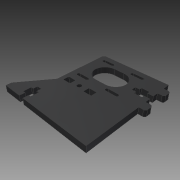
# Autodesk Inventor part: y_motor_mount
Saved by Autodesk Inventor 2014 (Build 180170000, 170)
## iProperties
Created: 2013-12-07
Part Number: y_motor_mount
Material: Generic
Document SubType Name: Modeling
Designer: buben
Density: 1 g/cm^3
Appearance: Anodized - Dark Gray
Author: buben
Subject: Laser Cutted
Autodesk Inventor part; units mm, degrees
ref_plane "YZ Plane" through (0, 0, 0) normal (1, 0, 0) x (0, 1, 0)
ref_plane "XZ Plane" through (0, 0, 0) normal (0, 1, 0) x (-1, 0, 0)
ref_plane "XY Plane" through (0, 0, 0) normal (0, 0, 1) x (1, 0, 0)
sketch "Sketch1" plane through (0, 0, 0) normal (0, 0, 1) x (1, 0, 0)
  line L0 (0, 0) -> (67.3, 0)
  line L1 (67.3, 0) -> (67.3, 55)
  line L2 (67.3, 55) -> (0, 55)
  line L3 (0, 55) -> (0, 0)
  line L4 (7, 48) -> (38, 48) construction
  line L5 (38, 48) -> (38, 17) construction
  line L6 (38, 17) -> (7, 17) construction
  line L7 (7, 17) -> (7, 48) construction
  line L8 (7, 48) -> (17, 48) construction
  line L9 (7, 49.6) -> (17, 49.6)
  line L10 (17, 46.4) -> (7, 46.4)
  arc A0 (7, 49.6) -> (7, 46.4) centre (7, 48) ccw
  arc A1 (17, 46.4) -> (17, 49.6) centre (17, 48) ccw
  line L11 (7, 17) -> (17, 17) construction
  line L12 (7, 18.6) -> (17, 18.6)
  line L13 (17, 15.4) -> (7, 15.4)
  arc A2 (7, 18.6) -> (7, 15.4) centre (7, 17) ccw
  arc A3 (17, 15.4) -> (17, 18.6) centre (17, 17) ccw
  line L14 (38, 48) -> (48, 48) construction
  line L15 (38, 46.4) -> (48, 46.4)
  line L16 (48, 49.6) -> (38, 49.6)
  arc A4 (38, 49.6) -> (38, 46.4) centre (38, 48) ccw
  arc A5 (48, 46.4) -> (48, 49.6) centre (48, 48) ccw
  line L17 (38, 17) -> (48, 17) construction
  line L18 (38, 18.6) -> (48, 18.6)
  line L19 (48, 15.4) -> (38, 15.4)
  arc A6 (38, 18.6) -> (38, 15.4) centre (38, 17) ccw
  arc A7 (48, 15.4) -> (48, 18.6) centre (48, 17) ccw
  line L20 (22.5, 32.5) -> (32.5, 32.5) construction
  line L21 (22.5, 44) -> (32.5, 44)
  line L22 (32.5, 21) -> (22.5, 21)
  arc A8 (22.5, 44) -> (22.5, 21) centre (22.5, 32.5) ccw
  arc A9 (32.5, 21) -> (32.5, 44) centre (32.5, 32.5) ccw
  point P0 (12, 48)
  point P1 (12, 17)
  point P2 (43, 48)
  point P3 (43, 17)
  point P4 (27.5, 32.5)
  point P5 (22.5, 48)
  point P6 (7, 32.5)
  dimension "d0" = 31
  dimension "d2" = 10
  dimension "d3" = 3.2
  dimension "d4" = 10
  dimension "d5" = 23
  dimension "d6" = 7
  dimension "d7" = 7
  dimension "d8" = 17
  dimension "d9" = 34.8
  constraints: 56 end point, 20 point on circle, 20 tangent, 14 parallel, 10 centre point, 7 midpoint, 6 coincident, 4 equal length, 3 equal radius, 3 horizontal alignment, 2 horizontal, 2 perpendicular, 1 vertical alignment
  measures "d0" distance of L5.end L6.end
  measures "d2" distance of L11.start L11.end
  measures "d3" distance between parallel lines of L13 L12
  measures "d4" distance of L20.start L20.end
  measures "d5" distance between parallel lines of L22 L21
  measures "d6" distance between parallel lines of L8 L2
  measures "d7" distance between parallel lines of L3 L7
  measures "d8" distance between parallel lines of L0 L6
  measures "d9" distance from line of L20.end L1
extrude "Extrusion1" add sketch "Sketch1" along normal blind 6
sketch "Sketch2" plane through (0, 0, 6) normal (0, 0, 1) x (1, 0, 0)
  line L0 (0, 0) -> (67.3, 0) projected
  line L1 (0, 55) -> (0, 0) projected
  line L2 (4, 9) -> (12, 9)
  line L3 (12, 9) -> (12, 3)
  line L4 (12, 3) -> (4, 3)
  line L5 (4, 3) -> (4, 9)
  line L6 (27, 9) -> (35, 9)
  line L7 (35, 9) -> (35, 3)
  line L8 (35, 3) -> (27, 3)
  line L9 (27, 3) -> (27, 9)
  line L10 (12, 3) -> (27, 9) construction
  line L11 (27, 3) -> (12, 9) construction
  circle A0 centre (19.5, 6) radius 2.25
  dimension "d12" = 8
  dimension "d13" = 6
  dimension "d14" = 15
  dimension "d15" = 4.5
  dimension "d16" = 3
  dimension "d17" = 4
  dimension "d18" = 8
  constraints: 20 end point, 4 parallel, 2 collinear, 2 horizontal, 2 perpendicular, 1 centre point, 1 midpoint
  measures "d12" distance of L2.start L2.end
  measures "d13" distance of L4.end L2.start
  measures "d14" distance between parallel lines of L9 L3
  measures "d15" diameter of A0
  measures "d16" distance between parallel lines of L0 L4
  measures "d17" distance between parallel lines of L1 L5
  measures "d18" distance of L6.start L6.end
extrude "Extrusion2" cut sketch "Sketch2" against normal blind 6
sketch "Sketch3" plane through (0, 0, 6) normal (0, 0, 1) x (1, 0, 0)
  arc A0 (32.5, 21) -> (32.5, 44) centre (32.5, 32.5) ccw projected
  line L0 (67.3, 0) -> (67.3, 55) projected
  line L1 (67.3, 34.75) -> (67.3, 30.25)
  line L2 (51, 30.25) -> (51, 34.75)
  line L3 (55, 37.25) -> (62.3, 37.25)
  line L4 (62.3, 27.75) -> (55, 27.75)
  line L5 (51, 34.75) -> (55, 34.75)
  line L6 (62.3, 34.75) -> (67.3, 34.75)
  line L7 (67.3, 30.25) -> (62.3, 30.25)
  line L8 (55, 30.25) -> (51, 30.25)
  line L9 (55, 27.75) -> (55, 30.25)
  line L10 (55, 34.75) -> (55, 37.25)
  line L11 (62.3, 37.25) -> (62.3, 34.75)
  line L12 (62.3, 30.25) -> (62.3, 27.75)
  point P0 (51, 32.5)
  dimension "d21" = 4.5
  dimension "d22" = 4
  dimension "d23" = 5
  dimension "d24" = 7.3
  dimension "d25" = 2.5
  dimension "d26" = 2.5
  constraints: 24 end point, 10 parallel, 5 collinear, 4 perpendicular, 3 horizontal, 1 horizontal alignment, 1 midpoint
  measures "d21" distance of L2.start L2.end
  measures "d22" distance of L2.end L5.end
  measures "d23" distance of L6.start L1.start
  measures "d24" distance of L3.start L3.end
  measures "d25" distance of L5.end L3.start
  measures "d26" distance of L4.end L8.start
extrude "Extrusion3" cut sketch "Sketch3" against normal blind 6
sketch "Sketch4" plane through (0, 0, 6) normal (0, 0, 1) x (1, 0, 0)
  line L0 (67.3, 34.75) -> (67.3, 55) projected
  line L1 (67.3, 0) -> (67.3, 30.25) projected
  line L2 (51, 30.25) -> (51, 34.75) projected
  line L3 (67.3, 40) -> (71.3, 40)
  line L4 (73.3, 42) -> (73.3, 46)
  line L5 (71.3, 48) -> (67.3, 48)
  line L6 (67.3, 48) -> (67.3, 40)
  line L7 (67.3, 25) -> (71.3, 25)
  line L8 (73.3, 23) -> (73.3, 19)
  line L9 (71.3, 17) -> (67.3, 17)
  line L10 (67.3, 17) -> (67.3, 25)
  arc A0 (73.3, 46) -> (71.3, 48) centre (71.3, 46) ccw
  arc A1 (71.3, 40) -> (73.3, 42) centre (71.3, 42) ccw
  arc A2 (73.3, 23) -> (71.3, 25) centre (71.3, 23) ccw
  arc A3 (71.3, 17) -> (73.3, 19) centre (71.3, 19) ccw
  point P0 (51, 32.5)
  dimension "d29" = 2
  dimension "d30" = 8
  dimension "d31" = 8
  dimension "d32" = 6
  dimension "d33" = 15
  dimension "d34" = 7.5
  constraints: 16 end point, 8 point on circle, 8 tangent, 4 centre point, 4 parallel, 3 equal radius, 2 horizontal, 2 perpendicular, 2 point on line, 1 collinear, 1 midpoint
  measures "d29" radius of A0
  measures "d30" distance between parallel lines of L5 L3
  measures "d31" distance between parallel lines of L9 L7
  measures "d32" distance between parallel lines of L0 L4
  measures "d33" distance between parallel lines of L7 L3
  measures "d34" distance from line of point (51, 32.5) L3
extrude "Extrusion4" add sketch "Sketch4" against normal blind 6
chamfer "Chamfer1" distance 2 angle 45 1 edges at (0, 55, 3)
sketch "Sketch5" plane through (0, 0, 6) normal (0, 0, 1) x (1, 0, 0)
  line L0 (7, 49.6) -> (17, 49.6) projected
  line L1 (-20.7, -33.49) -> (67.3, -33.49)
  line L2 (67.3, -33.49) -> (67.3, 0)
  line L3 (0, 0) -> (67.3, 0)
  line L4 (-20.7, -33.49) -> (-20.7, -28.49)
  line L5 (-20.7, -28.49) -> (0, 0)
  point P0 (67.3, 55)
  dimension "d40" = 88.49
  dimension "d41" = 88
  dimension "d42" = 5
  constraints: 10 end point, 3 perpendicular, 1 parallel
  measures "d40" distance of point (67.3, 55) L1.end
  measures "d41" distance of L1.start L1.end
  measures "d42" distance of L1.start L4.end
extrude "Extrusion5" add sketch "Sketch5" against normal blind 6
sketch "Sketch6" plane through (0, 0, 6) normal (0, 0, 1) x (1, 0, 0)
  line L0 (-20.7, -33.49) -> (67.3, -33.49) projected
  line L1 (-2.25, -17.19) -> (2.25, -17.19)
  line L2 (2.25, -33.49) -> (-2.25, -33.49)
  line L3 (4.75, -21.19) -> (4.75, -28.49)
  line L4 (-4.75, -28.49) -> (-4.75, -21.19)
  line L5 (-4.75, -21.19) -> (-2.25, -21.19)
  line L6 (2.25, -21.19) -> (4.75, -21.19)
  line L7 (4.75, -28.49) -> (2.25, -28.49)
  line L8 (-2.25, -28.49) -> (-4.75, -28.49)
  line L9 (-2.25, -33.49) -> (-2.25, -28.49)
  line L10 (-2.25, -21.19) -> (-2.25, -17.19)
  line L11 (2.25, -17.19) -> (2.25, -21.19)
  line L12 (2.25, -28.49) -> (2.25, -33.49)
  point P0 (0, 0)
  point P1 (0, -17.19)
  dimension "d45" = 4.5
  dimension "d46" = 2.5
  dimension "d47" = 2.5
  dimension "d48" = 5
  dimension "d49" = 4
  dimension "d50" = 7.3
  constraints: 24 end point, 10 parallel, 5 collinear, 4 perpendicular, 3 horizontal, 1 midpoint, 1 vertical alignment
  measures "d45" distance of L1.start L1.end
  measures "d46" distance of L4.end L5.end
  measures "d47" distance of L6.start L3.start
  measures "d48" distance of L2.end L8.start
  measures "d49" distance of L5.end L1.start
  measures "d50" distance of L4.start L4.end
extrude "Extrusion6" cut sketch "Sketch6" against normal blind 6
body "Solid1"
